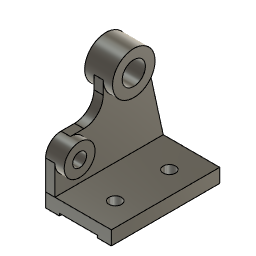
Sketch14_Final v1 (Autodesk Fusion 360 design; units mm, degrees)
Autodesk Fusion 360 part; units mm, degrees
sketch "Sketch1" plane through (0, 0, 0) normal (0, 1, 0) x (1, 0, 0)
  line L0 (-42.5, -18) -> (42.5, -18)
  line L1 (42.5, -18) -> (42.5, 0)
  line L2 (-42.5, 0) -> (-42.5, -18)
  line L3 (-42.5, 0) -> (-24.5, 0)
  line L4 (42.5, 0) -> (24.5, 0)
  line L5 (24.5, 0) -> (24.5, -3)
  line L6 (-24.5, 0) -> (-24.5, -3)
  line L7 (-24.5, -3) -> (24.5, -3)
  line L8 (-42.5, 0) -> (-24.5, 0)
  line L9 (24.5, 0) -> (42.5, 0)
  dimension "d40" = 18
  dimension "d41" = 18
  dimension "d42" = 49
  dimension "d43" = 3
  dimension "d44" = 18
  dimension "d45" = 85
  dimension "d46" = 3
  measures "d40" distance of L2.start L3.end
  measures "d41" distance of L1.end L4.end
  measures "d42" distance of L5.end L6.end
  measures "d43" distance of L4.end L5.end
  measures "d44" distance of L0.end L1.end
  measures "d45" distance of L0.start L0.end
  measures "d46" distance of L3.end L6.end
extrude "Extrude1" add sketch "Sketch1" along normal blind 140 makes body 1
sketch "Sketch2" plane through (0, 0, 18) normal (0, 0, 1) x (-1, 0, 0)
  line L0 (42.5, 0) -> (-42.5, 0)
  line L1 (-42.5, 0) -> (-42.5, -140)
  line L2 (-42.5, -140) -> (42.5, -140)
  line L3 (42.5, -140) -> (42.5, 0)
  line L4 (42.5, -140) -> (30.5, -140)
  line L5 (30.5, 0) -> (42.5, 0)
  line L6 (42.5, 0) -> (42.5, -140)
  circle A0 centre (-12.5, -35) radius 8
  circle A1 centre (-12.5, -105) radius 8
  line L7 (42.5, 0) -> (30.5, 0)
  line L8 (30.5, 0) -> (30.5, -140)
  line L9 (30.5, -140) -> (42.5, -140)
  line L10 (42.5, -140) -> (42.5, 0)
  dimension "d14" = 12
  dimension "d15" = 140
  constraint horizontal L4
  constraint horizontal L5
  constraint vertical L6
  constraint coincident L2.end L3.start
  constraint horizontal L7
  constraint vertical L8
  constraint horizontal L9
  constraint vertical L10
  constraint coincident L0.start L3.end
  measures "d14" distance of L0.start L5.start
  measures "d15" distance of L0.start L2.end
extrude "Extrude2" cut sketch "Sketch2" against normal blind 20 contours A0 | A1 bodies 1
sketch "Sketch3" plane through (0, 0, 0) normal (1, 0, 0) x (0, 1, 0)
  line L0 (140, 18) -> (0, 18)
  line L1 (0, 18) -> (0, 56)
  line L2 (0, 18) -> (20, 18)
  circle A0 centre (20, 56) radius 20
  line L3 (140, 18) -> (90, 18)
  circle A1 centre (90, 118) radius 15
  circle A2 centre (90, 118) radius 27.5
  line L4 (20, 76) -> (37.5, 76)
  line L5 (62.5, 101) -> (62.5, 118)
  arc A3 (37.5, 76) -> (62.5, 101) centre (37.5, 101) ccw
  line L6 (140, 18) -> (116.8661, 123.8705)
  circle A4 centre (20, 56) radius 9
  dimension "d20" = 140
  dimension "d22" = 20
  dimension "d23" = 38
  dimension "d24" = 40
  dimension "d25" = 50
  dimension "d29" = 25
  dimension "d30" = 18
  constraint horizontal L0
  constraint vertical L1
  constraint perpendicular L1 L2
  constraint concentric A1 A2
  constraint coincident A0 L4.start
  constraint tangent A0 L4
  constraint coincident A2 L5.end
  constraint tangent L4 A3
  constraint coincident A2 L6.end
  constraint tangent A2 L6
  constraint coincident A0 L1.end
  constraint concentric A0 A4
  measures "d20" distance of L0.start L0.end
  measures "d22" distance of L0.end L2.end
  measures "d23" distance of L2.end A0.centre
  measures "d24" diameter of A0
  measures "d25" distance of L0.start L3.end
  measures "d29" radius of A3
  measures "d30" diameter of A4
extrude "Extrude4" add sketch "Sketch3" along normal blind 12 from surface at -42.5 separate body makes body 2
extrude "Extrude5" add sketch "Sketch3" along normal blind 24 from surface at -42.5 contours A0 bodies 2
extrude "Extrude6" add sketch "Sketch3" along normal mid plane 36 from surface at -36.5 contours A2 bodies 2
